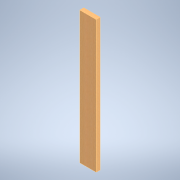
# Autodesk Inventor part: wooden beams
Saved by Autodesk Inventor 2021 (Build 250183000, 183)
## iProperties
Created: 2020-09-19
Part Number: wooden beams
Material: Wood (Oak)
Document SubType Name: Modeling
Designer: Jawad
Density: 0.76 g/cm^3
Appearance: Yellow Pine - Solid Stained Dark No Gloss
Author: Jawad
Autodesk Inventor part; units mm, degrees
ref_plane "YZ Plane" through (0, 0, 0) normal (1, 0, 0) x (0, 1, 0)
ref_plane "XZ Plane" through (0, 0, 0) normal (0, 1, 0) x (-1, 0, 0)
ref_plane "XY Plane" through (0, 0, 0) normal (0, 0, 1) x (1, 0, 0)
sketch "floor beams" plane through (0, 0, 0) normal (0, 1, 0) x (-1, 0, 0)
  line L0 (143.1381, 46.3041) -> (-131.8619, 46.3041)
  line L1 (-131.8619, 46.3041) -> (-131.8619, -22.4459)
  line L2 (-131.8619, -22.4459) -> (143.1381, -22.4459)
  line L3 (143.1381, -22.4459) -> (143.1381, 46.3041)
  point P0 (0, 0)
  dimension "d0" = 68.75
  dimension "d1" = 275
  constraints: 8 end point, 2 parallel, 1 horizontal, 1 perpendicular
  measures "d0" distance of L2.end L0.start
  measures "d1" distance of L0.start L0.end
extrude "Extrusion1" add sketch "floor beams" along normal blind 2200
equation "\"d0\" = 0.25 * d1"
body "Solid1"
